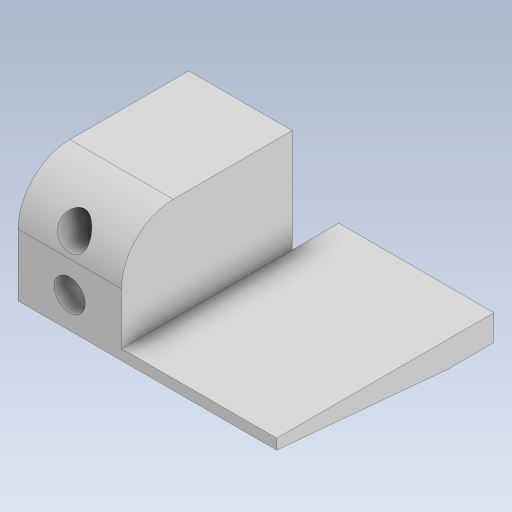
# Autodesk Inventor part: Holder Motor Lifter 2
Saved by Autodesk Inventor 2023.5 (Build 275446000, 446)
## iProperties
Created: 2025-09-06
Part Number: Holder Motor Lifter 2
Material: Generic
Document SubType Name: Modeling
Designer: Guntur
Density: 1 g/cm^3
Appearance: Default
Author: Guntur
Autodesk Inventor part; units mm, degrees
sketch "Sketch1" plane through (0, 0, 0) normal (0, 1, 0) x (-1, 0, 0)
  line L0 (0, 0) -> (-20, 0)
  line L1 (-20, 0) -> (-20, -13)
  line L2 (-20, -13) -> (0, -13)
  line L3 (0, -13) -> (0, 0)
  line L4 (0, -13) -> (20, -13)
  line L5 (20, -13) -> (20, -10)
  line L6 (20, -10) -> (0, -10)
  line L7 (0, -10) -> (0, -13)
  line L8 (0, -13) -> (-20, -13)
  line L9 (-20, -13) -> (-20, -23)
  line L10 (-20, -23) -> (0, -23)
  line L11 (0, -23) -> (0, -13)
  line L12 (20, -10) -> (0, -10)
  line L13 (0, -10) -> (0, 0)
  line L14 (0, 0) -> (20, 0)
  line L15 (20, 0) -> (20, -10)
  dimension "d0" = 20
  dimension "d1" = 13
  dimension "d2" = 20
  dimension "d3" = 3
  dimension "d4" = 10
  constraints: 32 end point, 8 parallel, 4 horizontal, 4 perpendicular
  measures "d0" distance of L2.end L1.end
  measures "d1" distance of L1.end L0.end
  measures "d2" distance of L6.end L5.end
  measures "d3" distance of L5.end L4.end
  measures "d4" distance of L9.end L8.end
extrude "Extrusion1" add sketch "Sketch1" along normal blind 2 contours L3 L2 L1 L0 | L2 L11 L10 L9
extrude "Extrusion2" add sketch "Sketch1" along normal blind 22 contours L6 L5 L4 L3
extrude "Extrusion3" add sketch "Sketch1" along normal blind 2 contours L14 L15 L6 L3
ref_plane "Work Plane1" through (-10, 2, -13) normal (1, 0, 0) x (0, 0, -1)
sketch "Sketch2" plane through (-10, 2, -13) normal (1, 0, 0) x (0, 0, -1)
  line L0 (0, 20) -> (-3, 20) projected
  line L1 (-13, -2) -> (-13, 0) projected
  line L2 (-13, 0) -> (-3, 0)
  line L3 (-3, 0) -> (-3, 20) projected
  line L4 (-3, 0) -> (-3, 20)
  line L5 (-3, 20) -> (-13, 20)
  line L6 (-13, 20) -> (-13, 0)
  line L7 (-13, 0) -> (-3, 0)
  line L8 (-3, 0) -> (-3, 20)
  constraints: 12 end point, 3 perpendicular, 2 parallel, 1 horizontal
extrude "Extrusion4" add sketch "Sketch2" along normal mid plane 20
fillet "Fillet1" radius 10 1 edges at (-10, 22, 0)
sketch "Sketch3" plane through (0, 0, -13) normal (0, 0, -1) x (-1, 0, 0)
  circle A0 centre (10, 16) radius 1.5
  line L0 (0, 22) -> (20, 22) projected
  circle A1 centre (10, 6) radius 1.5
  line L1 (0, 0) -> (20, 0) projected
  point P0 (10, 0)
  dimension "d14" = 3
  dimension "d15" = 6
  dimension "d16" = 3
  dimension "d18" = 6
  constraints: 2 centre point, 1 midpoint
  measures "d14" diameter of A0
  measures "d15" distance from line of L0 A0.centre
  measures "d16" diameter of A1
  measures "d18" distance of point (10, 0) A1.centre
extrude "Extrusion5" cut sketch "Sketch3" against normal blind 20
ref_plane "Work Plane2" through (0, 0, -6.5) normal (0, 0, -1) x (-1, 0, 0)
sketch "Sketch4" plane through (0, 0, -6.5) normal (0, 0, -1) x (-1, 0, 0)
  circle A0 centre (10, 16) radius 1.5 projected
  circle A1 centre (10, 16) radius 3
  circle A2 centre (10, 6) radius 1.5 projected
  circle A3 centre (10, 6) radius 3
  point P0 (0, 0)
  dimension "d21" = 6
  dimension "d22" = 6
  constraints: 2 centre point, 2 coincident
  measures "d21" diameter of A1
  measures "d22" diameter of A3
extrude "Extrusion6" cut sketch "Sketch4" against normal blind 20
sketch "Sketch5" plane through (0, 0, -13) normal (0, 0, -1) x (-1, 0, 0)
  line L0 (0, 22) -> (20, 22) projected
  line L1 (0, 0) -> (20, 0) projected
  line L2 (0, 22) -> (20, 22)
  line L3 (20, 22) -> (20, 0)
  line L4 (20, 0) -> (0, 0)
  line L5 (0, 0) -> (0, 22)
  circle A0 centre (10, 16) radius 1.5 projected
  circle A1 centre (10, 16) radius 1.5
  circle A2 centre (10, 6) radius 1.5 projected
  circle A3 centre (10, 6) radius 1.5
  constraints: 8 end point, 2 centre point, 2 coincident, 2 parallel, 1 horizontal, 1 perpendicular
extrude "Extrusion7" add sketch "Sketch5" along normal blind 10
ref_plane "Work Plane3" through (0, 0, 0) normal (1, 0, 0) x (0, 0, -1)
sketch "Sketch6" plane through (0, 0, 0) normal (1, 0, 0) x (0, 0, -1)
  line L0 (0, 0) -> (23, 0) projected
  line L1 (23, 0) -> (23, -2)
  line L2 (23, -2) -> (0, 0)
  line L3 (0, 0) -> (23, 0)
  dimension "d27" = 2
  constraints: 6 end point, 1 collinear, 1 vertical
  measures "d27" distance of L0.end L1.end
extrude "Extrusion8" add sketch "Sketch6" along normal mid plane 40
sketch "Sketch7" plane through (0, 22, -23) normal (0, 0, -1) x (-1, 0, 0)
  line L0 (20, 0) -> (0, 0) projected
  line L1 (20, -24) -> (20, -22) projected
  line L2 (0, 0) -> (20, 0)
  line L3 (20, 0) -> (20, -24)
  line L4 (20, -24) -> (0, -24)
  line L5 (0, -24) -> (0, 0)
  line L6 (0, -20) -> (-20, -20) projected
  line L7 (-20, -20) -> (0, -20)
  line L8 (0, -20) -> (0, -24)
  line L9 (0, -24) -> (-20, -24)
  line L10 (-20, -24) -> (-20, -20)
  circle A0 centre (10, -6) radius 1.5 projected
  circle A1 centre (10, -6) radius 1.5
  circle A2 centre (10, -16) radius 1.5 projected
  circle A3 centre (10, -16) radius 1.5
  point P0 (0, -22)
  constraints: 16 end point, 4 parallel, 2 centre point, 2 coincident, 2 horizontal, 2 perpendicular
extrude "Extrusion9" add sketch "Sketch7" along normal blind 10
sketch "Sketch8" plane through (0, 0, 0) normal (1, 0, 0) x (0, 0, -1)
  line L0 (23, -2) -> (33, -2) projected
  line L1 (33, -2) -> (33, -3)
  line L2 (33, -3) -> (23, -2)
  point P0 (0, 0)
  dimension "d32" = 1
  constraints: 4 end point, 1 vertical
  measures "d32" distance of L0.end L1.end
extrude "Extrusion10" add sketch "Sketch8" along normal mid plane 40
sketch "Sketch9" plane through (20, 0, 0) normal (1, 0, 0) x (0, 0, -1)
  line L0 (33, 2) -> (0, 2) projected
  line L1 (0, 2) -> (33, 2)
  line L2 (33, 2) -> (33, -3) projected
  line L3 (33, 2) -> (33, -3)
  line L4 (23, -2) -> (0, 0) projected
  line L5 (33, -3) -> (0, 0)
  line L6 (0, 0) -> (0, 2)
  constraints: 8 end point, 1 collinear, 1 horizontal
extrude "Extrusion11" add sketch "Sketch9" along normal blind 10
sketch "Sketch10" plane through (0, 22, -33) normal (0, 0, -1) x (-1, 0, 0)
  line L0 (0, -20) -> (-30, -20) projected
  line L1 (-30, -20) -> (0, -20)
  line L2 (0, -20) -> (0, -25)
  line L3 (-20, -25) -> (20, -25) projected
  line L4 (-30, -25) -> (-30, -20) projected
  line L5 (-30, -25) -> (-30, -20)
  line L6 (-20, -24) -> (-20, -25) projected
  line L7 (-20, -25) -> (-30, -25) projected
  line L8 (-20, -25) -> (-30, -25)
  point P0 (0, -22)
  constraints: 8 end point, 3 collinear, 1 midpoint
extrude "Extrusion12" add sketch "Sketch10" along normal blind 9
body "Solid1"
